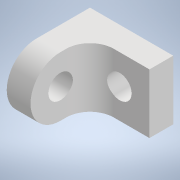
# Autodesk Inventor part: conector 90°
Saved by Autodesk Inventor 2020 (Build 240168000, 168)
## iProperties
Created: 2020-04-22
Part Number: conector 90°
Material: Genérico
Document SubType Name: Modeling
Designer: gi-se
Density: 1 g/cm^3
Appearance: Padrão
Author: gi-se
Autodesk Inventor part; units mm, degrees
ref_plane "YZ Plane" through (0, 0, 0) normal (1, 0, 0) x (0, 1, 0)
ref_plane "XZ Plane" through (0, 0, 0) normal (0, 1, 0) x (-1, 0, 0)
ref_plane "XY Plane" through (0, 0, 0) normal (0, 0, 1) x (1, 0, 0)
sketch "Esboço1" plane through (0, 0, 0) normal (0, 1, 0) x (-1, 0, 0)
  line L0 (66, 0) -> (59, 0)
  line L1 (59, 0) -> (59, 2)
  line L2 (59, 2) -> (62, 2)
  line L3 (66, 2) -> (66, 0)
  line L4 (66, 0) -> (64, 0)
  line L5 (64, 4) -> (64, 7)
  line L6 (64, 7) -> (66, 7)
  line L7 (66, 7) -> (66, 0)
  arc A0 (62, 2) -> (64, 4) centre (62, 4) ccw
  point P0 (0, 0)
  dimension "d0" = 2
  constraints: 16 end point, 4 parallel, 2 horizontal, 2 perpendicular, 2 point on circle, 2 tangent, 1 centre point
  measures "d0" radius of A0
extrude "Extrusão1" add sketch "Esboço1" along normal blind 5
sketch "Esboço2" plane through (-59, 0, 0) normal (0, 0, -1) x (-1, 0, 0)
  circle A0 centre (2.5, 2.5) radius 1
  line L0 (0, 0) -> (7, 0) projected
  line L1 (0, 0) -> (0, 5) projected
  arc A1 (2.5, 5) -> (2.5, 0) centre (2.5, 2.5) ccw
  line L2 (3, 0) -> (0, 0) projected
  line L3 (3, 5) -> (0, 5) projected
  line L4 (2.5, 0) -> (0, 0)
  line L5 (0, 0) -> (0, 5)
  line L6 (0, 5) -> (2.5, 5)
  point P0 (-59, 0)
  point P1 (0, 2.5)
  dimension "d3" = 2
  dimension "d4" = 2.5
  dimension "d5" = 2.5
  constraints: 6 end point, 2 centre point, 2 point on circle, 1 coincident, 1 horizontal, 1 parallel, 1 perpendicular, 1 point on line
  measures "d3" diameter of A0
  measures "d4" distance from line of L0 A0.centre
  measures "d5" distance from line of L1 A0.centre
extrude "Extrusão2" cut sketch "Esboço2" against normal blind 4.25
sketch "Esboço3" plane through (-66, 0, 0) normal (-1, 0, 0) x (0, 0, 1)
  circle A0 centre (4.5, 2.5) radius 1
  line L0 (0, 5) -> (7, 5) projected
  line L1 (7, 0) -> (7, 5) projected
  arc A1 (4.5, 0) -> (4.5, 5) centre (4.5, 2.5) ccw
  line L2 (7, 0) -> (4, 0) projected
  line L3 (7, 5) -> (4, 5) projected
  line L4 (4.5, 0) -> (7, 0)
  line L5 (7, 0) -> (7, 5)
  line L6 (7, 5) -> (4.5, 5)
  point P0 (0, 0)
  point P1 (4.5, 5)
  point P2 (7, 2.5)
  dimension "d8" = 2.5
  dimension "d9" = 2.5
  constraints: 6 end point, 2 centre point, 2 point on circle, 1 coincident, 1 horizontal, 1 parallel, 1 perpendicular, 1 point on line
  measures "d8" distance from line of L0 A0.centre
  measures "d9" distance from line of L1 A0.centre
extrude "Extrusão3" cut sketch "Esboço3" against normal blind 4.25
sketch "Esboço4" plane through (-66, 0, 0) normal (0, 0, -1) x (-1, 0, 0)
  line L0 (0, -91.1) -> (0, 5) projected
  line L1 (-4.5, 0) -> (0, 0) projected
  line L2 (-4.5, 5) -> (0, 5) projected
  point P0 (-66, 0)
